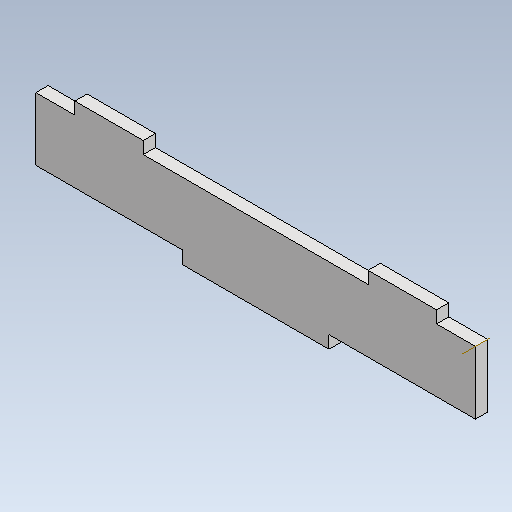
# Autodesk Inventor part: lower-front-back-plate-support
Saved by Autodesk Inventor 2025 (Build 290162000, 162)
## iProperties
Created: 2025-08-21
Part Number: lower-front-back-plate-support
Material: Generic
Document SubType Name: Modeling
Designer: HP
Density: 1 g/cm^3
Appearance: Default
Author: HP
Autodesk Inventor part; units mm, degrees
ref_plane "YZ Plane" through (0, 0, 0) normal (1, 0, 0) x (0, 1, 0)
ref_plane "XZ Plane" through (0, 0, 0) normal (0, 1, 0) x (-1, 0, 0)
ref_plane "XY Plane" through (0, 0, 0) normal (0, 0, 1) x (1, 0, 0)
sketch "Sketch1" plane through (0, 0, 0) normal (0, 0, 1) x (1, 0, 0)
  line L0 (-90, -18) -> (90, -18)
  line L1 (90, -18) -> (90, 18)
  line L2 (90, 18) -> (-90, 18)
  line L3 (-90, 18) -> (-90, -18)
  line L4 (-90, -18) -> (90, 18) construction
  line L5 (90, -18) -> (-90, 18) construction
  line L6 (-46.05, 18) -> (46.05, 18)
  line L7 (46.05, 18) -> (46.05, 13)
  line L8 (46.05, 13) -> (-46.05, 13)
  line L9 (-46.05, 13) -> (-46.05, 18)
  line L10 (-46.05, 18) -> (46.05, 13) construction
  line L11 (46.05, 18) -> (-46.05, 13) construction
  line L12 (-90, -12.8) -> (-30, -12.8)
  line L13 (-30, -12.8) -> (-30, -18)
  line L14 (-30, -18) -> (-90, -18)
  line L15 (-90, -18) -> (-90, -12.8)
  line L16 (-90, -12.8) -> (-30, -18) construction
  line L17 (-30, -12.8) -> (-90, -18) construction
  line L18 (19.6182, -18) -> (70, -18)
  line L19 (0, 0) -> (0, -18) construction
  line L20 (30, -18) -> (90, -18)
  line L21 (90, -18) -> (90, -12.8)
  line L22 (90, -12.8) -> (30, -12.8)
  line L23 (30, -12.8) -> (30, -18)
  line L24 (30, -18) -> (90, -12.8) construction
  line L25 (90, -18) -> (30, -12.8) construction
  line L26 (-45.85, 18) -> (-74.05, 18)
  line L27 (74.05, 18) -> (74.05, 13)
  line L28 (74.05, 13) -> (90, 13)
  line L29 (-74.05, 18) -> (-74.05, 13)
  line L30 (-74.05, 13) -> (-90, 13)
  point P0 (0, 15.5)
  point P1 (-60, -15.4)
  point P2 (46.05, 18)
  point P3 (-46.05, 18)
  point P4 (-30, -18)
  point P5 (-90, -12.8)
  point P6 (60, -15.4)
  point P7 (30, -18)
  point P8 (-74.05, 18)
  dimension "d0" = 180
  dimension "d1" = 36
  dimension "d10" = 5
  dimension "d11" = 92.1
  dimension "d12" = 5.2
  dimension "d21" = 5.2
  dimension "d24" = 60
  dimension "d31" = 28
  dimension "d32" = 28
  constraints: 62 end point, 9 midpoint, 8 collinear, 8 parallel, 6 horizontal, 5 perpendicular, 3 point on line, 1 vertical alignment, 1 other
  measures "d0" distance between parallel lines of L1 L3
  measures "d1" distance between parallel lines of L0 L2
  measures "d10" distance between parallel lines of L8 L6
  measures "d11" distance between parallel lines of L9 L7
  measures "d12" distance between parallel lines of L14 L12
  measures "d21" distance between parallel lines of L20 L22
  measures "d24" distance between parallel lines of L23 L13
  measures "d31" distance between parallel lines of L7 L27
  measures "d32" distance between parallel lines of L9 L29
extrude "Extrusion1" add sketch "Sketch1" along normal blind 5 contours L13 L12 L3 L30 L29 L2 L9 L8 L7 L27 L28 L1 L22 L23 L0
equation "\"d32\" = d31"
body "Solid1"
